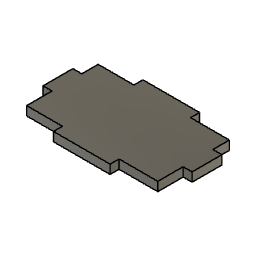
NEW Spool (Autodesk Fusion 360 design; units mm, degrees)
Autodesk Fusion 360 part; units mm, degrees
sketch "Sketch1" plane through (0, 0, 0) normal (0, 0, 1) x (1, 0, 0)
  line L0 (50, 125) -> (62, 125)
  line L1 (62, 125) -> (62, 128)
  line L2 (62, 128) -> (81, 128)
  line L3 (81, 128) -> (81, 125)
  line L4 (81, 125) -> (94, 125)
  line L5 (94, 125) -> (94, 119.5)
  line L6 (94, 119.5) -> (97, 119.5)
  line L7 (97, 119.5) -> (97, 109.5)
  line L8 (97, 109.5) -> (94, 109.5)
  line L9 (94, 109.5) -> (94, 101)
  line L10 (94, 101) -> (81, 101)
  line L11 (81, 101) -> (81, 98)
  line L12 (81, 98) -> (62, 98)
  line L13 (62, 98) -> (62, 101)
  line L14 (62, 101) -> (50, 101)
  line L15 (50, 101) -> (50, 109.5)
  line L16 (50, 109.5) -> (47, 109.5)
  line L17 (47, 109.5) -> (47, 119.5)
  line L18 (47, 119.5) -> (50, 119.5)
  line L19 (50, 119.5) -> (50, 125)
  dimension "d1" = 12
  dimension "d2" = 3
  dimension "d3" = 19
  dimension "d4" = 3
  dimension "d5" = 13
  dimension "d6" = 5.5
  dimension "d7" = 3
  dimension "d8" = 10
  dimension "d9" = 3
  dimension "d10" = 8.5
  dimension "d11" = 13
  dimension "d12" = 3
  dimension "d13" = 19
  dimension "d14" = 3
  dimension "d15" = 12
  dimension "d16" = 8.5
  dimension "d17" = 3
  dimension "d18" = 10
  dimension "d19" = 3
  constraint horizontal L0
  constraint perpendicular L0 L1
  constraint perpendicular L1 L2
  constraint perpendicular L0 L3
  constraint perpendicular L3 L4
  constraint perpendicular L0 L5
  constraint perpendicular L3 L6
  constraint perpendicular L0 L7
  constraint perpendicular L3 L8
  constraint perpendicular L8 L9
  constraint perpendicular L3 L10
  constraint perpendicular L10 L11
  constraint perpendicular L3 L12
  constraint perpendicular L10 L13
  constraint perpendicular L3 L14
  constraint perpendicular L10 L15
  constraint perpendicular L3 L16
  constraint perpendicular L10 L17
  constraint perpendicular L3 L18
  measures "d1" distance of L0.start L0.end
  measures "d2" distance of L0.end L1.end
  measures "d3" distance of L1.end L2.end
  measures "d4" distance of L2.end L3.end
  measures "d5" distance of L3.end L4.end
  measures "d6" distance of L4.end L5.end
  measures "d7" distance of L5.end L6.end
  measures "d8" distance of L6.end L7.end
  measures "d9" distance of L7.end L8.end
  measures "d10" distance of L8.end L9.end
  measures "d11" distance of L9.end L10.end
  measures "d12" distance of L10.end L11.end
  measures "d13" distance of L11.end L12.end
  measures "d14" distance of L12.end L13.end
  measures "d15" distance of L13.end L14.end
  measures "d16" distance of L14.end L15.end
  measures "d17" distance of L15.end L16.end
  measures "d18" distance of L16.end L17.end
  measures "d19" distance of L17.end L18.end
extrude "Extrude1" add sketch "Sketch1" along normal blind 3
